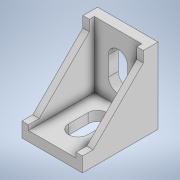
# Autodesk Inventor part: 3030_angle
Saved by Autodesk Inventor 2022 (Build 260153000, 153)
## iProperties
Created: 2022-06-18
Part Number: 3030_angle
Material: Generic
Document SubType Name: Modeling
Designer: logic
Density: 1 g/cm^3
Appearance: Default
Author: logic
Autodesk Inventor part; units mm, degrees
ref_plane "YZ Plane" through (0, 0, 0) normal (1, 0, 0) x (0, 1, 0)
ref_plane "XZ Plane" through (0, 0, 0) normal (0, 1, 0) x (-1, 0, 0)
ref_plane "XY Plane" through (0, 0, 0) normal (0, 0, 1) x (1, 0, 0)
sketch "Sketch1" plane through (0, 0, 0) normal (0, 1, 0) x (-1, 0, 0)
  line L0 (14, 17.5) -> (-14, 17.5)
  line L1 (-14, 17.5) -> (-14, -17.5)
  line L2 (-14, -17.5) -> (14, -17.5)
  line L3 (14, -17.5) -> (14, 17.5)
  point P0 (0, 0)
  dimension "d0" = 35
  dimension "d1" = 28
  dimension "d2" = 14
  dimension "d3" = 17.5
  constraints: 8 end point, 2 parallel, 1 horizontal, 1 perpendicular
  measures "d0" distance of L0.end L1.end
  measures "d1" distance of L1.end L2.end
  measures "d2" distance from line of point (0, 0) L3
  measures "d3" distance from line of L2 point (0, 0)
extrude "Extrusion1" add sketch "Sketch1" along normal blind 4.5
sketch "Sketch2" plane through (14, 0, 17.5) normal (1, 0, 0) x (0, 0, -1)
  line L0 (0, 0) -> (35, 0) projected
  line L1 (35, 0) -> (35, 4.5) projected
  line L2 (0, 4.5) -> (35, 4.5) projected
  line L3 (0, 0) -> (0, 4.5) projected
  line L4 (35, 0) -> (35, 35)
  line L5 (35, 35) -> (28.2, 35)
  line L6 (28.2, 35) -> (28.2, 30)
  line L7 (28.2, 30) -> (5, 6.8)
  line L8 (5, 6.8) -> (0, 6.8)
  line L9 (0, 0) -> (35, 0) projected
  line L10 (0, 6.8) -> (0, 0)
  point P0 (17.5, 0)
  point P1 (0, 4.5)
  dimension "d6" = 6.8
  dimension "d7" = 5
  constraints: 12 end point, 5 perpendicular, 2 vertical, 1 parallel
  measures "d6" distance of L8.end L0.start
  measures "d7" distance of L5.end L6.end
extrude "Extrusion2" add sketch "Sketch2" against normal blind 3 contours L10 L8 L7 L6 L5 L4 L2
sketch "Sketch3" plane through (-14, 0, -17.5) normal (-1, 0, 0) x (0, 0, 1)
  line L0 (35, 4.5) -> (35, 6.8) projected
  line L1 (35, 6.8) -> (30, 6.8) projected
  line L2 (30, 6.8) -> (6.8, 30) projected
  line L3 (6.8, 30) -> (6.8, 35) projected
  line L4 (6.8, 35) -> (0, 35) projected
  line L5 (0, 35) -> (0, 4.5) projected
  line L6 (35, 4.5) -> (0, 4.5) projected
  line L7 (0, 0) -> (35, 0) projected
  line L8 (35, 0) -> (35, 4.5) projected
  line L9 (0, 4.5) -> (35, 4.5) projected
  line L10 (0, 0) -> (0, 4.5) projected
  point P0 (17.5, 0)
  point P1 (0, 4.5)
extrude "Extrusion3" add sketch "Sketch3" against normal blind 3
sketch "Sketch4" plane through (14, 0, -17.5) normal (0, 0, -1) x (-1, 0, 0)
  line L0 (3, 4.5) -> (25, 4.5) projected
  line L1 (3, 35) -> (3, 4.5) projected
  line L2 (0, 35) -> (3, 35) projected
  line L3 (0, 0) -> (0, 35) projected
  line L4 (0, 0) -> (28, 0) projected
  line L5 (28, 0) -> (28, 35) projected
  line L6 (28, 35) -> (25, 35) projected
  line L7 (25, 4.5) -> (25, 35) projected
  line L8 (0, 35) -> (3, 35) projected
  line L9 (28, 30) -> (28, 35) projected
  line L10 (0, 35) -> (28, 35)
  point P0 (14, 0)
  point P1 (25, 35)
  constraints: 2 end point, 1 horizontal
extrude "Extrusion4" add sketch "Sketch4" against normal blind 4.5
sketch "Sketch5" plane through (0, 4.5, 0) normal (0, 1, 0) x (1, 0, 0)
  line L0 (14, -17.5) -> (14, 17.5) projected
  line L1 (-14, -17.5) -> (14, -17.5) projected
  line L2 (-14, 17.5) -> (-14, -17.5) projected
  line L3 (14, 17.5) -> (-14, 17.5) projected
  line L4 (11, 13) -> (-11, 13) projected
  line L5 (-11, 13) -> (-11, -17.5) projected
  line L6 (-11, -17.5) -> (11, -17.5) projected
  line L7 (11, -17.5) -> (11, 13) projected
  line L8 (0, 3.5) -> (0, -5.5) construction
  line L9 (-4.4, 3.5) -> (-4.4, -5.5)
  line L10 (4.4, -5.5) -> (4.4, 3.5)
  arc A0 (4.4, 3.5) -> (-4.4, 3.5) centre (0, 3.5) ccw
  arc A1 (-4.4, -5.5) -> (4.4, -5.5) centre (0, -5.5) ccw
  point P0 (0, 0)
  point P1 (0, -1)
  dimension "d14" = 14
  dimension "d15" = 9
  dimension "d16" = 8.8
  constraints: 8 end point, 4 point on circle, 4 tangent, 2 centre point, 1 midpoint, 1 parallel, 1 point on line, 1 vertical
  measures "d14" distance from line of L8.start L3
  measures "d15" distance of L8.end L8.start
  measures "d16" distance between parallel lines of L10 L9
extrude "Extrusion5" cut sketch "Sketch5" against normal through all contours A0 L10 A1 L9
sketch "Sketch6" plane through (14, 0, -13) normal (0, 0, 1) x (1, 0, 0)
  line L0 (-14, 23) -> (-14, 14) construction
  line L1 (-18.4, 23) -> (-18.4, 14)
  line L2 (-9.6, 14) -> (-9.6, 23)
  arc A0 (-9.6, 23) -> (-18.4, 23) centre (-14, 23) ccw
  arc A1 (-18.4, 14) -> (-9.6, 14) centre (-14, 14) ccw
  line L3 (-28, 0) -> (0, 0) projected
  line L4 (-14, 7.4113) -> (0, 7.4113) construction
  line L5 (0, 30) -> (0, 6.8) projected
  point P0 (-14, 0)
  point P1 (-14, 18.5)
  dimension "d19" = 9
  dimension "d20" = 8.8
  dimension "d21" = 14
  dimension "d22" = 14
  constraints: 10 end point, 4 point on circle, 4 tangent, 2 centre point, 2 point on line, 1 horizontal, 1 midpoint, 1 parallel, 1 vertical
  measures "d19" distance of L0.end L0.start
  measures "d20" distance between parallel lines of L2 L1
  measures "d21" distance from line of L3 L0.end
  measures "d22" distance of L4.start L4.end
extrude "Extrusion6" cut sketch "Sketch6" against normal blind 10
body "Solid1"
